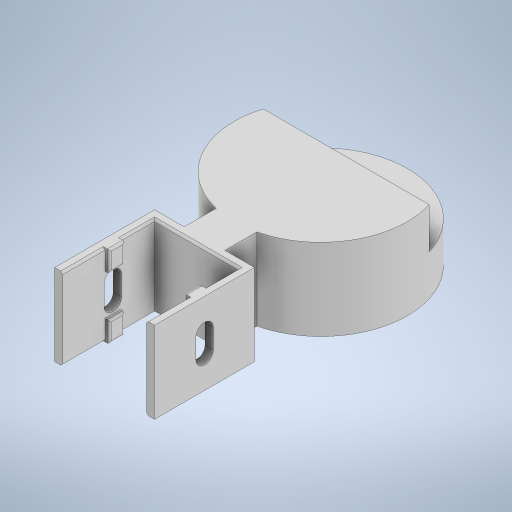
# Autodesk Inventor part: Bi_PAM_top_slot2
Saved by Autodesk Inventor 2024 (Build 280153000, 153)
## iProperties
Created: 2023-07-27
Part Number: Bi_PAM_top_slot2
Material: 일반
Document SubType Name: Modeling
Designer: jsw
Density: 1 g/cm^3
Appearance: 기본값
Author: jsw
Autodesk Inventor part; units mm, degrees
ref_plane "YZ Plane" through (0, 0, 0) normal (1, 0, 0) x (0, 1, 0)
ref_plane "XZ Plane" through (0, 0, 0) normal (0, 1, 0) x (-1, 0, 0)
sketch "스케치1" plane through (0, 0, 0) normal (0, 1, 0) x (-1, 0, 0)
  circle A0 centre (0, 0) radius 39
  circle A1 centre (0, 0) radius 42.5
  dimension "d0" = 78
  dimension "d1" = 3.5
  constraints: 2 centre point, 2 coincident
  measures "d0" diameter of A0
  measures "d1" radial gap between concentric circles of A0 A1
extrude "돌출1" add sketch "스케치1" along normal blind 7 contours A0 | A1
sketch "스케치2" plane through (0, 0, 0) normal (0, -1, 0) x (1, 0, 0)
  line L0 (15, -36.2132) -> (-15, -36.2132)
  line L1 (-15, -36.2132) -> (-36.2132, -15)
  line L2 (-36.2132, -15) -> (-36.2132, 15)
  line L3 (-36.2132, 15) -> (-15, 36.2132)
  line L4 (-15, 36.2132) -> (15, 36.2132)
  line L5 (15, 36.2132) -> (36.2132, 15)
  line L6 (36.2132, 15) -> (36.2132, -15)
  line L7 (36.2132, -15) -> (15, -36.2132)
  point P0 (0, 0)
  point P1 (0, 0)
  dimension "d5" = 30
  constraints: 16 end point, 1 coincident, 1 horizontal, 17 other
  measures "d5" distance of L5.end L6.end
extrude "돌출2" cut sketch "스케치2" against normal blind 4
fillet "모깎기1" radius 1.2 8 edges at (0, 4, 36.2132) (-25.6066, 4, 25.6066) (25.6066, 4, 25.6066) (36.2132, 4, 0) (25.6066, 4, -25.6066) (0, 4, -36.2132) (-25.6066, 4, -25.6066) (-36.2132, 4, 0)
sketch "스케치3" plane through (0, 0, 0) normal (0, -1, 0) x (1, 0, 0)
  line L0 (-15, 36.2132) -> (15, 36.2132) projected
  circle A0 centre (0, 0) radius 39.1969
  circle A1 centre (0, 0) radius 41.1969
  dimension "d9" = 2
  constraints: 2 coincident, 1 centre point, 3 other
extrude "돌출3" cut sketch "스케치3" against normal blind 4
sketch "스케치4" plane through (0, 7, 0) normal (0, 1, 0) x (1, 0, 0)
  line L0 (-15, 12.5) -> (15, 12.5)
  line L1 (15, 12.5) -> (15, -12.5)
  line L2 (15, -12.5) -> (-15, -12.5)
  line L3 (-15, -12.5) -> (-15, 12.5)
  point P0 (0, 0)
  point P1 (0, 12.5)
  point P2 (15, 0)
  dimension "d12" = 30
  dimension "d13" = 25
  constraints: 8 end point, 2 midpoint, 2 parallel, 1 horizontal, 1 horizontal alignment, 1 perpendicular, 1 vertical alignment
  measures "d12" distance of L0.start L0.end
  measures "d13" distance of L0.end L1.end
extrude "돌출4" add sketch "스케치4" along normal blind 20
sketch "스케치6" plane through (0, 4, 0) normal (0, -1, 0) x (1, 0, 0)
  line L0 (10.5, -7.75) -> (-10.5, -7.75)
  line L1 (-10.5, -7.75) -> (-10.5, -2.25)
  line L2 (-10.5, -2.25) -> (10.5, -2.25)
  line L3 (10.5, -2.25) -> (10.5, -7.75)
  line L4 (10.5, -7.75) -> (-10.5, -2.25) construction
  line L5 (-10.5, -7.75) -> (10.5, -2.25) construction
  line L6 (0, 0) -> (-35.0132, 0)
  line L7 (-35.0132, -14.5029) -> (-35.0132, 14.5029) projected
  line L8 (10.5, 7.75) -> (-10.5, 7.75)
  line L9 (-10.5, 7.75) -> (-10.5, 2.25)
  line L10 (-10.5, 2.25) -> (10.5, 2.25)
  line L11 (10.5, 2.25) -> (10.5, 7.75)
  line L12 (10.5, 7.75) -> (-10.5, 2.25) construction
  line L13 (-10.5, 7.75) -> (10.5, 2.25) construction
  point P0 (0, -5)
  point P1 (10.5, -5)
  point P2 (0, 5)
  point P3 (10.5, 5)
  dimension "d18" = 21
  dimension "d19" = 5.5
  dimension "d76" = 5
  constraints: 26 end point, 6 symmetric about line, 4 midpoint, 2 parallel, 1 horizontal, 1 perpendicular, 1 vertical alignment
  measures "d18" distance of L1.end L2.end
  measures "d19" distance of L0.end L1.end
  measures "d76" distance of point (0, -5) L6.start
extrude "돌출5" cut sketch "스케치6" against normal blind 12
sketch "스케치10" plane through (0, 0, 0) normal (0, -1, 0) x (1, 0, 0)
  circle A0 centre (0, 0) radius 41.1969 projected
  circle A1 centre (0, 0) radius 42.5 projected
extrude "돌출9" add sketch "스케치10" along normal blind 13
sketch "스케치11" plane through (0, 7, 0) normal (0, 1, 0) x (1, 0, 0)
  line L0 (-10, -61) -> (10, -61)
  line L1 (10, -61) -> (10, -41)
  line L2 (10, -41) -> (-10, -41)
  line L3 (-10, -41) -> (-10, -61)
  line L4 (-10, -61) -> (10, -41) construction
  line L5 (10, -61) -> (-10, -41) construction
  circle A0 centre (0, 0) radius 42.5 projected
  point P0 (0, -51)
  point P1 (10, -41.3068)
  point P2 (-10, -41.3068)
  dimension "d44" = 10
  dimension "d45" = 20
  dimension "d49" = 41
  constraints: 12 end point, 2 midpoint, 2 parallel, 1 horizontal, 1 perpendicular, 1 vertical alignment
  measures "d44" distance from line of point (0, -51) L1
  measures "d45" distance of L0.end L1.end
  measures "d49" distance from line of L2 point (0, 0)
extrude "돌출10" add sketch "스케치11" along normal mid plane 40 contours L3 A0 L1 L0
sketch "스케치12" plane through (0, 7, 0) normal (0, 1, 0) x (1, 0, 0)
  line L0 (20.5, -102) -> (-20.5, -102)
  line L1 (-20.5, -102) -> (-20.5, -61)
  line L2 (-20.5, -61) -> (20.5, -61)
  line L3 (20.5, -61) -> (20.5, -102)
  line L4 (20.5, -102) -> (-20.5, -61) construction
  line L5 (-20.5, -102) -> (20.5, -61) construction
  line L6 (24.5, -106) -> (-24.5, -106)
  line L7 (-24.5, -106) -> (-24.5, -57)
  line L8 (-24.5, -57) -> (24.5, -57)
  line L9 (24.5, -57) -> (24.5, -106)
  line L10 (24.5, -106) -> (-24.5, -57) construction
  line L11 (-24.5, -106) -> (24.5, -57) construction
  line L12 (10, -61) -> (-10, -61) projected
  line L13 (-20.5, -102) -> (-20.5, -106)
  line L14 (20.5, -102) -> (20.5, -106)
  point P0 (0, 0)
  point P1 (0, -81.5)
  point P2 (0, -61)
  dimension "d50" = 41
  dimension "d51" = 41
  dimension "d52" = 4
  dimension "d53" = 20.5
  constraints: 28 end point, 5 midpoint, 4 parallel, 4 perpendicular, 3 point on line, 2 horizontal, 1 vertical alignment
  measures "d50" distance of L1.end L2.end
  measures "d51" distance of L2.end L0.start
  measures "d52" distance between parallel lines of L2 L8
  measures "d53" distance of point (0, -61) point (0, -81.5)
extrude "돌출11" add sketch "스케치12" along normal mid plane 40 contours L3 L2 L1 L13 L6 L7 L8 L9 L14
sketch "스케치13" plane through (-24.5, -13, 57) normal (-1, 0, 0) x (0, 0, -1)
  line L0 (-24.5, -15.25) -> (-24.5, -24.75) construction
  line L1 (-28.75, -15.25) -> (-28.75, -24.75)
  line L2 (-20.25, -24.75) -> (-20.25, -15.25)
  arc A0 (-20.25, -15.25) -> (-28.75, -15.25) centre (-24.5, -15.25) ccw
  arc A1 (-28.75, -24.75) -> (-20.25, -24.75) centre (-24.5, -24.75) ccw
  line L3 (-49, 0) -> (0, 0) projected
  point P0 (57, -13)
  point P1 (-24.5, -20)
  point P2 (-24.5, -29)
  point P3 (-24.5, -11)
  point P4 (-20.25, -20)
  point P5 (-24.5, 0)
  point P6 (-24.5, 0)
  dimension "d56" = 18
  dimension "d57" = 4.25
  dimension "d58" = 20
  constraints: 8 end point, 6 point on circle, 4 midpoint, 4 tangent, 2 centre point, 1 parallel, 1 vertical, 1 vertical alignment
  measures "d56" distance of point (-24.5, -29) point (-24.5, -11)
  measures "d57" distance of point (-24.5, -20) point (-20.25, -20)
  measures "d58" distance of point (-24.5, 0) point (-24.5, -20)
extrude "돌출12" cut sketch "스케치13" against normal up to surface (49 mm away)
sketch "스케치14" plane through (20.5, -13, 61) normal (-1, 0, 0) x (0, 0, -1)
  line L0 (-45, 0) -> (0, 0) projected
  line L1 (-24.25, 0) -> (-16.75, 0)
  line L2 (-16.75, 0) -> (-16.75, -10)
  line L3 (-16.75, -10) -> (-24.25, -10)
  line L4 (-24.25, -10) -> (-24.25, 0)
  arc A0 (-16.25, -15.25) -> (-24.75, -15.25) centre (-20.5, -15.25) ccw projected
  line L5 (-24.75, -24.75) -> (-24.75, -15.25) projected
  line L6 (-24.75, -20) -> (-16.25, -20)
  line L7 (-16.25, -15.25) -> (-16.25, -24.75) projected
  line L8 (0, -40) -> (-45, -40)
  line L9 (-24.25, -40) -> (-16.75, -40)
  line L10 (-16.75, -40) -> (-16.75, -30)
  line L11 (-16.75, -30) -> (-24.25, -30)
  line L12 (-24.25, -30) -> (-24.25, -40)
  point P0 (61, -13)
  point P1 (-20.5, 0)
  point P2 (-20.5, -11)
  point P3 (-20.5, -40)
  point P4 (-16.75, -40)
  point P5 (-16.75, 0)
  dimension "d61" = 7.5
  dimension "d62" = 10
  constraints: 20 end point, 7 symmetric about line, 3 midpoint, 2 parallel, 2 point on line, 1 horizontal, 1 perpendicular, 1 point on circle, 1 vertical alignment
  measures "d61" distance of L2.end L3.end
  measures "d62" distance of L1.end L2.end
extrude "돌출13" add sketch "스케치14" along normal blind 2 contours L0 L2 L3 L4 | L8 L12 L11 L10
fillet "모깎기2" radius 1 8 edges at (18.5, -13, 81.5) (18.5, -8, 85.25) (18.5, -8, 77.75) (18.5, -3, 81.5) (18.5, 17, 81.5) (18.5, 22, 77.75) (18.5, 27, 81.5) (18.5, 22, 85.25)
ref_plane "작업 평면1" through (0, 27, 106) normal (-1, 0, 0) x (0, 0, 1)
mirror "미러1" about plane through (0, 27, 106) normal (-1, 0, 0) of "모깎기2", "돌출13"
chamfer "모따기2" distance 1 angle 45 10 edges at (20.5, -13, 95.625) (20.5, -13, 69.375) (-20.5, -13, 69.375) (-20.5, -13, 95.625) (0, -13, 61) (0, 27, 61) (20.5, 27, 95.625) (20.5, 27, 69.375) (-20.5, 27, 69.375) (-20.5, 27, 95.625)
sketch "스케치15" plane through (0, 7, 0) normal (0, 1, 0) x (1, 0, 0)
  line L0 (15, 12.5) -> (15, -12.5) projected
  arc A0 (-10, -41.3068) -> (10, -41.3068) centre (0, 0) ccw projected
  line L1 (15, -12.5) -> (10, -41.3068)
  line L2 (10, -41.3068) -> (-10, -41.3068)
  line L3 (-15, 12.5) -> (-15, -12.5) projected
  line L4 (-10, -41.3068) -> (-15, -12.5)
  line L5 (-15, -12.5) -> (15, -12.5)
  line L6 (-15, 12.5) -> (15, 12.5) projected
  line L7 (-15, 12.5) -> (-40.6202, 12.5)
  line L8 (15, 12.5) -> (40.6202, 12.5)
  arc A1 (10, -41.3068) -> (-10, -41.3068) centre (0, 0) ccw projected
  constraints: 12 end point, 2 horizontal, 2 point on circle, 1 perpendicular
extrude "돌출14" add sketch "스케치15" along normal up to surface (20 mm away) contours L8 A1 L1 L0 | L1 L2 L4 L5 | L3 L4 A1 L7 | A0 L2
chamfer "모따기4" distance 1 angle 45 8 edges at (0, 4, 7.75) (-10.5, 4, 5) (0, 4, 2.25) (10.5, 4, 5) (10.5, 4, -5) (0, 4, -2.25) (-10.5, 4, -5) (0, 4, -7.75)
sketch "스케치16" plane through (40.6202, 7, -12.5) normal (0, 0, -1) x (-1, 0, 0)
  circle A0 centre (45.6202, 5) radius 1.25
  line L0 (81.2404, 0) -> (0, 0) projected
  line L1 (40.6202, 0) -> (40.6202, 20)
  line L2 (81.2404, 20) -> (0, 20) projected
  circle A1 centre (35.6202, 5) radius 1.25
  point P0 (40.6202, -7)
  dimension "d80" = 2.5
  dimension "d81" = 5
  dimension "d82" = 10
  constraints: 2 centre point, 2 end point, 2 midpoint, 1 symmetric about line, 1 other
  measures "d80" diameter of A0
  measures "d81" distance from line of A0.centre L0
  measures "d82" distance of A1.centre A0.centre
extrude "돌출15" cut sketch "스케치16" against normal blind 25
equation "\"d53\" = 0.5 * d51"
